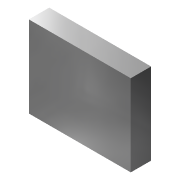
# Autodesk Inventor part: suporte-barra
Saved by Autodesk Inventor 2015 (Build 190159000, 159)
## iProperties
Created: 2016-08-11
Part Number: suporte-barra
Material: Steel, Carbon
Document SubType Name: Modeling
Designer: EriveltonDell
Density: 7.87 g/cm^3
Appearance: Chrome - Polished
Mass: 377.778 g
Surface Area: 137.801 cm^2
Volume: 48.0022 cm^3
Author: EriveltonDell
Autodesk Inventor part; units mm, degrees
ref_plane "YZ Plane" through (0, 0, 0) normal (1, 0, 0) x (0, 1, 0)
ref_plane "XZ Plane" through (0, 0, 0) normal (0, 1, 0) x (-1, 0, 0)
ref_plane "XY Plane" through (0, 0, 0) normal (0, 0, 1) x (1, 0, 0)
sketch "Sketch11" plane through (0, 0, 0) normal (0, 1, 0) x (-1, 0, 0)
  line L0 (0, 0) -> (50, 0)
  line L1 (50, 0) -> (50, 40)
  line L2 (50, 40) -> (0, 40)
  line L3 (0, 40) -> (0, 0)
  dimension "d63" = 50
  dimension "d64" = 40
  constraints: 8 end point, 2 parallel, 1 horizontal, 1 perpendicular
  measures "d63" distance of L2.end L1.end
  measures "d64" distance of L1.end L0.end
extrude "Extrusion10" add sketch "Sketch11" along normal blind 10
body "Solid2"
